Autodesk Fusion 360 part; units mm, degrees
note: some values were not read from the file. Chosen so that the rebuilt part matches the saved one: which bodies a step acts on; which face or edge a step refers to. Set by a fixed rule: which sketch regions a step uses.
(part 2 of 3)
  constraint collinear L37 L38
  constraint collinear L39 L40
  constraint coincident L41.end L43
  constraint collinear L41 L42
  constraint coincident L43.end L113
  constraint collinear L43 L44
  constraint collinear L45 L46
  constraint collinear L47 L48
  constraint coincident L50.start L55
  constraint collinear L49 L50
  constraint coincident L52.start L53
  constraint collinear L51 L52
  constraint collinear L53 L54
  constraint collinear L55 L56
  constraint coincident L58.start L59
  constraint collinear L57 L58
  constraint collinear L59 L60
  constraint coincident L62.start L111
  constraint collinear L61 L62
  constraint collinear L63 L64
  constraint coincident L65.end L67
  constraint collinear L65 L66
  constraint coincident L67.end L71
  constraint collinear L67 L68
  constraint collinear L69 L70
  constraint collinear L71 L72
  constraint collinear L73 L74
  constraint coincident L76.start L81
  constraint collinear L75 L76
  constraint coincident L78.start L79
  constraint collinear L77 L78
  constraint collinear L79 L80
  constraint collinear L81 L82
  constraint coincident L84.start L89
  constraint collinear L83 L84
  constraint coincident L86.start L109
  constraint collinear L85 L86
  constraint collinear L87 L88
  constraint collinear L89 L90
  constraint coincident L91.end L95
  constraint collinear L91 L92
  constraint collinear L93 L94
  constraint coincident L95.end L99
  constraint collinear L95 L96
  constraint collinear L97 L98
  constraint collinear L99 L100
  constraint coincident L102.start L107
  constraint collinear L101 L102
  constraint coincident L104.start L105
  constraint collinear L103 L104
  constraint collinear L105 L106
  constraint collinear L107 L108
  constraint collinear L109 L110
  constraint collinear L111 L112
  constraint collinear L113 L114
  constraint perpendicular L35 L115
  constraint perpendicular L36 L116
  constraint collinear L341 L342
  constraint coincident L344.start L349
  constraint collinear L343 L344
  constraint coincident L346.start L347
  constraint collinear L345 L346
  constraint collinear L347 L348
  constraint collinear L349 L350
  constraint coincident L351.end L355
  constraint collinear L351 L352
  constraint collinear L353 L354
  constraint coincident L355.end L367
  constraint collinear L355 L356
  constraint coincident L358.start L365
  constraint collinear L357 L358
  constraint coincident L360.start L361
  constraint collinear L359 L360
  constraint coincident A101.end L361
  constraint collinear L361 L362
  constraint collinear L363 L364
  constraint collinear L365 L366
  constraint collinear L367 L368
  constraint coincident L370.start L375
  constraint collinear L369 L370
  constraint coincident L372.start L373
  constraint collinear L371 L372
  constraint collinear L373 L374
  constraint collinear L375 L376
  constraint collinear L377 L378
  constraint coincident L379.end L383
  constraint collinear L379 L380
  constraint coincident L381.end L385
  constraint collinear L381 L382
  constraint collinear L383 L384
  constraint collinear L385 L386
  constraint collinear L387 L388
  constraint coincident L388.start L395
  constraint collinear L389 L390
  constraint coincident L392.start L393
  constraint collinear L391 L392
  constraint collinear L393 L394
  constraint collinear L395 L396
  constraint coincident L398.start L403
  constraint collinear L397 L398
  constraint coincident L400.start L401
  constraint collinear L399 L400
  constraint collinear L401 L402
  constraint collinear L403 L404
  constraint coincident L405.end L409
  constraint collinear L405 L406
  constraint collinear L407 L408
  constraint coincident L409.end L413
  constraint collinear L409 L410
  constraint collinear L411 L412
  constraint collinear L413 L414
  constraint coincident L416.start L423
  constraint collinear L415 L416
  constraint coincident L418.start L421
  constraint collinear L417 L418
  constraint collinear L419 L420
  constraint collinear L421 L422
  constraint collinear L423 L424
  measures "d74" distance of L342.end L352.end
  measures "d82" distance of L341 L355
  measures "d88" diameter of A100
  measures "d89" diameter of A99
  measures "d93" distance of L349 L367
  measures "d95" distance of L341.start L342.end
  measures "d98" distance of A100.centre L367
  measures "d103" distance of L341 L343
  measures "d104" diameter of A97
  measures "d105" diameter of A98
  measures "d106" diameter of A96
  measures "d107" distance of A96.centre L341
  measures "d113" distance of L3.start L3.end
move_body "Sposta4" bodies 1 to x (1, 0, 0) y (0, 1, 0) z (0, 0, 1) at (-120, 0, 0) in component "Cubo"
extrude "Estrusione10" cut sketch "Schizzo14" against normal blind 10 bodies 2 in component "Cubo"
fillet "Raccordo2" radius 2 4 edges at (86, 4, 13.5) (86, 86, 13.5) (4, 4, 13.5) (4, 86, 13.5) on bodies 2 in component "Cubo"
sketch "Schizzo17" plane through (0, 0, 16) normal (0, 0, 1) x (-1, 0, 0) in component "Cubo"
  line L0 (-47.5456, -19.25) -> (-48.649, -19.25)
  arc A0 (-48.649, -18.05) -> (-48.649, -19.25) centre (-49.7456, -18.65) ccw
  line L1 (-48.649, -18.05) -> (-47.5456, -18.05)
  line L2 (-47.5456, -18.05) -> (-47.5456, -12.5)
  line L3 (-47.5456, -12.5) -> (-46.2956, -12.5)
  line L4 (-46.2956, -12.5) -> (-46.2956, -10.9)
  line L5 (-46.2956, -10.9) -> (-48.649, -10.9)
  arc A1 (-48.649, -9.7) -> (-48.649, -10.9) centre (-49.7456, -10.3) ccw
  line L6 (-48.649, -9.7) -> (-46.2956, -9.7)
  line L7 (-46.2956, -9.7) -> (-46.2956, -8.9715)
  arc A2 (-43.6956, -8.9715) -> (-46.2956, -8.9715) centre (-44.9956, -7.8) ccw
  line L8 (-43.6956, -8.9715) -> (-43.6956, -9.7)
  line L9 (-43.6956, -9.7) -> (-41.3421, -9.7)
  arc A3 (-41.3421, -10.9) -> (-41.3421, -9.7) centre (-40.2456, -10.3) ccw
  line L10 (-41.3421, -10.9) -> (-43.6956, -10.9)
  line L11 (-43.6956, -10.9) -> (-43.6956, -12.5)
  line L12 (-43.6956, -12.5) -> (-42.4456, -12.5)
  line L13 (-42.4456, -12.5) -> (-42.4456, -18.05)
  line L14 (-42.4456, -18.05) -> (-41.3421, -18.05)
  arc A4 (-41.3421, -19.25) -> (-41.3421, -18.05) centre (-40.2456, -18.65) ccw
  line L15 (-41.3421, -19.25) -> (-42.4456, -19.25)
  line L16 (-42.4456, -19.25) -> (-42.4456, -24.8)
  line L17 (-42.4456, -24.8) -> (-43.6956, -24.8)
  line L18 (-43.6956, -24.8) -> (-43.6956, -26.4)
  line L19 (-43.6956, -26.4) -> (-41.3421, -26.4)
  arc A5 (-41.3421, -27.6) -> (-41.3421, -26.4) centre (-40.2456, -27) ccw
  line L20 (-41.3421, -27.6) -> (-43.6956, -27.6)
  line L21 (-43.6956, -27.6) -> (-43.6956, -28.3285)
  arc A6 (-46.2956, -28.3285) -> (-43.6956, -28.3285) centre (-44.9956, -29.5) ccw
  line L22 (-46.2956, -28.3285) -> (-46.2956, -27.6)
  line L23 (-46.2956, -27.6) -> (-48.649, -27.6)
  arc A7 (-48.649, -26.4) -> (-48.649, -27.6) centre (-49.7456, -27) ccw
  line L24 (-48.649, -26.4) -> (-46.2956, -26.4)
  line L25 (-46.2956, -26.4) -> (-46.2956, -24.8)
  line L26 (-46.2956, -24.8) -> (-47.5456, -24.8)
  line L27 (-47.5456, -24.8) -> (-47.5456, -19.25)
  arc A8 (-27.7171, -37.25) -> (-27.7171, -36.05) centre (-26.6206, -36.65) ccw
  line L28 (-27.7171, -37.25) -> (-30.0706, -37.25)
  line L29 (-30.0706, -37.25) -> (-30.0706, -38.85)
  line L30 (-30.0706, -38.85) -> (-28.8206, -38.85)
  line L31 (-28.8206, -38.85) -> (-28.8206, -44.4)
  line L32 (-28.8206, -44.4) -> (-27.7171, -44.4)
  arc A9 (-27.7171, -45.6) -> (-27.7171, -44.4) centre (-26.6206, -45) ccw
  line L33 (-27.7171, -45.6) -> (-28.8206, -45.6)
  line L34 (-28.8206, -45.6) -> (-28.8206, -51.15)
  line L35 (-28.8206, -51.15) -> (-30.0706, -51.15)
  line L36 (-30.0706, -51.15) -> (-30.0706, -52.75)
  line L37 (-30.0706, -52.75) -> (-27.7171, -52.75)
  arc A10 (-27.7171, -53.95) -> (-27.7171, -52.75) centre (-26.6206, -53.35) ccw
  line L38 (-27.7171, -53.95) -> (-30.0706, -53.95)
  line L39 (-30.0706, -53.95) -> (-30.0706, -54.6785)
  arc A11 (-32.6706, -54.6785) -> (-30.0706, -54.6785) centre (-31.3706, -55.85) ccw
  line L40 (-32.6706, -54.6785) -> (-32.6706, -53.95)
  line L41 (-32.6706, -53.95) -> (-35.024, -53.95)
  arc A12 (-35.024, -52.75) -> (-35.024, -53.95) centre (-36.1206, -53.35) ccw
  line L42 (-35.024, -52.75) -> (-32.6706, -52.75)
  line L43 (-32.6706, -52.75) -> (-32.6706, -51.15)
  line L44 (-32.6706, -51.15) -> (-33.9206, -51.15)
  line L45 (-33.9206, -51.15) -> (-33.9206, -45.6)
  line L46 (-33.9206, -45.6) -> (-35.024, -45.6)
  arc A13 (-35.024, -44.4) -> (-35.024, -45.6) centre (-36.1206, -45) ccw
  line L47 (-35.024, -44.4) -> (-33.9206, -44.4)
  line L48 (-33.9206, -44.4) -> (-33.9206, -38.85)
  line L49 (-33.9206, -38.85) -> (-32.6706, -38.85)
  line L50 (-32.6706, -38.85) -> (-32.6706, -37.25)
  line L51 (-32.6706, -37.25) -> (-35.024, -37.25)
  arc A14 (-35.024, -36.05) -> (-35.024, -37.25) centre (-36.1206, -36.65) ccw
  line L52 (-35.024, -36.05) -> (-32.6706, -36.05)
  line L53 (-32.6706, -36.05) -> (-32.6706, -35.3215)
  arc A15 (-30.0706, -35.3215) -> (-32.6706, -35.3215) centre (-31.3706, -34.15) ccw
  line L54 (-30.0706, -35.3215) -> (-30.0706, -36.05)
  line L55 (-30.0706, -36.05) -> (-27.7171, -36.05)
  line L56 (-70.9456, -79.1) -> (-68.5921, -79.1)
  arc A16 (-68.5921, -80.3) -> (-68.5921, -79.1) centre (-67.4956, -79.7) ccw
  line L57 (-68.5921, -80.3) -> (-70.9456, -80.3)
  line L58 (-70.9456, -80.3) -> (-70.9456, -81.0285)
  arc A17 (-73.5456, -81.0285) -> (-70.9456, -81.0285) centre (-72.2456, -82.2) ccw
  line L59 (-73.5456, -81.0285) -> (-73.5456, -80.3)
  line L60 (-73.5456, -80.3) -> (-75.899, -80.3)
  arc A18 (-75.899, -79.1) -> (-75.899, -80.3) centre (-76.9956, -79.7) ccw
  line L61 (-75.899, -79.1) -> (-73.5456, -79.1)
  line L62 (-73.5456, -79.1) -> (-73.5456, -77.5)
  line L63 (-73.5456, -77.5) -> (-74.7956, -77.5)
  line L64 (-74.7956, -77.5) -> (-74.7956, -71.95)
  line L65 (-74.7956, -71.95) -> (-75.899, -71.95)
  arc A19 (-75.899, -70.75) -> (-75.899, -71.95) centre (-76.9956, -71.35) ccw
  line L66 (-75.899, -70.75) -> (-74.7956, -70.75)
  line L67 (-74.7956, -70.75) -> (-74.7956, -65.2)
  line L68 (-74.7956, -65.2) -> (-73.5456, -65.2)
  line L69 (-73.5456, -65.2) -> (-73.5456, -63.6)
  line L70 (-73.5456, -63.6) -> (-75.899, -63.6)
  arc A20 (-75.899, -62.4) -> (-75.899, -63.6) centre (-76.9956, -63) ccw
  line L71 (-75.899, -62.4) -> (-73.5456, -62.4)
  line L72 (-73.5456, -62.4) -> (-73.5456, -61.6715)
  arc A21 (-70.9456, -61.6715) -> (-73.5456, -61.6715) centre (-72.2456, -60.5) ccw
  line L73 (-70.9456, -61.6715) -> (-70.9456, -62.4)
  line L74 (-70.9456, -62.4) -> (-68.5921, -62.4)
  arc A22 (-68.5921, -63.6) -> (-68.5921, -62.4) centre (-67.4956, -63) ccw
  line L75 (-68.5921, -63.6) -> (-70.9456, -63.6)
  line L76 (-70.9456, -63.6) -> (-70.9456, -65.2)
  line L77 (-70.9456, -65.2) -> (-69.6956, -65.2)
  line L78 (-69.6956, -65.2) -> (-69.6956, -70.75)
  line L79 (-69.6956, -70.75) -> (-68.5921, -70.75)
  arc A23 (-68.5921, -71.95) -> (-68.5921, -70.75) centre (-67.4956, -71.35) ccw
  line L80 (-68.5921, -71.95) -> (-69.6956, -71.95)
  line L81 (-69.6956, -71.95) -> (-69.6956, -77.5)
  line L82 (-69.6956, -77.5) -> (-70.9456, -77.5)
  line L83 (-70.9456, -77.5) -> (-70.9456, -79.1)
  line L84 (-15.1956, -70.75) -> (-14.0921, -70.75)
  arc A24 (-14.0921, -71.95) -> (-14.0921, -70.75) centre (-12.9956, -71.35) ccw
  line L85 (-14.0921, -71.95) -> (-15.1956, -71.95)
  line L86 (-15.1956, -71.95) -> (-15.1956, -77.5)
  line L87 (-15.1956, -77.5) -> (-16.4456, -77.5)
  line L88 (-16.4456, -77.5) -> (-16.4456, -79.1)
  line L89 (-16.4456, -79.1) -> (-14.0921, -79.1)
  arc A25 (-14.0921, -80.3) -> (-14.0921, -79.1) centre (-12.9956, -79.7) ccw
  line L90 (-14.0921, -80.3) -> (-16.4456, -80.3)
  line L91 (-16.4456, -80.3) -> (-16.4456, -81.0285)
  arc A26 (-19.0456, -81.0285) -> (-16.4456, -81.0285) centre (-17.7456, -82.2) ccw
  line L92 (-19.0456, -81.0285) -> (-19.0456, -80.3)
  line L93 (-19.0456, -80.3) -> (-21.399, -80.3)
  arc A27 (-21.399, -79.1) -> (-21.399, -80.3) centre (-22.4956, -79.7) ccw
  line L94 (-21.399, -79.1) -> (-19.0456, -79.1)
  line L95 (-19.0456, -79.1) -> (-19.0456, -77.5)
  line L96 (-19.0456, -77.5) -> (-20.2956, -77.5)
  line L97 (-20.2956, -77.5) -> (-20.2956, -71.95)
  line L98 (-20.2956, -71.95) -> (-21.399, -71.95)
  arc A28 (-21.399, -70.75) -> (-21.399, -71.95) centre (-22.4956, -71.35) ccw
  line L99 (-21.399, -70.75) -> (-20.2956, -70.75)
  line L100 (-20.2956, -70.75) -> (-20.2956, -65.2)
  line L101 (-20.2956, -65.2) -> (-19.0456, -65.2)
  line L102 (-19.0456, -65.2) -> (-19.0456, -63.6)
  line L103 (-19.0456, -63.6) -> (-21.399, -63.6)
  arc A29 (-21.399, -62.4) -> (-21.399, -63.6) centre (-22.4956, -63) ccw
  line L104 (-21.399, -62.4) -> (-19.0456, -62.4)
  line L105 (-19.0456, -62.4) -> (-19.0456, -61.6715)
  arc A30 (-16.4456, -61.6715) -> (-19.0456, -61.6715) centre (-17.7456, -60.5) ccw
  line L106 (-16.4456, -61.6715) -> (-16.4456, -62.4)
  line L107 (-16.4456, -62.4) -> (-14.0921, -62.4)
  arc A31 (-14.0921, -63.6) -> (-14.0921, -62.4) centre (-12.9956, -63) ccw
  line L108 (-14.0921, -63.6) -> (-16.4456, -63.6)
  line L109 (-16.4456, -63.6) -> (-16.4456, -65.2)
  line L110 (-16.4456, -65.2) -> (-15.1956, -65.2)
  line L111 (-15.1956, -65.2) -> (-15.1956, -70.75)
  line L112 (-57.3206, -62.4) -> (-54.9671, -62.4)
  arc A32 (-54.9671, -63.6) -> (-54.9671, -62.4) centre (-53.8706, -63) ccw
  line L113 (-54.9671, -63.6) -> (-57.3206, -63.6)
  line L114 (-57.3206, -63.6) -> (-57.3206, -65.2)
  line L115 (-57.3206, -65.2) -> (-56.0706, -65.2)
  line L116 (-56.0706, -65.2) -> (-56.0706, -70.75)
  line L117 (-56.0706, -70.75) -> (-54.9671, -70.75)
  arc A33 (-54.9671, -71.95) -> (-54.9671, -70.75) centre (-53.8706, -71.35) ccw
  line L118 (-54.9671, -71.95) -> (-56.0706, -71.95)
  line L119 (-56.0706, -71.95) -> (-56.0706, -77.5)
  line L120 (-56.0706, -77.5) -> (-57.3206, -77.5)
  line L121 (-57.3206, -77.5) -> (-57.3206, -79.1)
  line L122 (-57.3206, -79.1) -> (-54.9671, -79.1)
  arc A34 (-54.9671, -80.3) -> (-54.9671, -79.1) centre (-53.8706, -79.7) ccw
  line L123 (-54.9671, -80.3) -> (-57.3206, -80.3)
  line L124 (-57.3206, -80.3) -> (-57.3206, -81.0285)
  arc A35 (-59.9206, -81.0285) -> (-57.3206, -81.0285) centre (-58.6206, -82.2) ccw
  line L125 (-59.9206, -81.0285) -> (-59.9206, -80.3)
  line L126 (-59.9206, -80.3) -> (-62.274, -80.3)
  arc A36 (-62.274, -79.1) -> (-62.274, -80.3) centre (-63.3706, -79.7) ccw
  line L127 (-62.274, -79.1) -> (-59.9206, -79.1)
  line L128 (-59.9206, -79.1) -> (-59.9206, -77.5)
  line L129 (-59.9206, -77.5) -> (-61.1706, -77.5)
  line L130 (-61.1706, -77.5) -> (-61.1706, -71.95)
  line L131 (-61.1706, -71.95) -> (-62.274, -71.95)
  arc A37 (-62.274, -70.75) -> (-62.274, -71.95) centre (-63.3706, -71.35) ccw
  line L132 (-62.274, -70.75) -> (-61.1706, -70.75)
  line L133 (-61.1706, -70.75) -> (-61.1706, -65.2)
  line L134 (-61.1706, -65.2) -> (-59.9206, -65.2)
  line L135 (-59.9206, -65.2) -> (-59.9206, -63.6)
  line L136 (-59.9206, -63.6) -> (-62.274, -63.6)
  arc A38 (-62.274, -62.4) -> (-62.274, -63.6) centre (-63.3706, -63) ccw
  line L137 (-62.274, -62.4) -> (-59.9206, -62.4)
  line L138 (-59.9206, -62.4) -> (-59.9206, -61.6715)
  arc A39 (-57.3206, -61.6715) -> (-59.9206, -61.6715) centre (-58.6206, -60.5) ccw
  line L139 (-57.3206, -61.6715) -> (-57.3206, -62.4)
  line L140 (-47.5456, -45.6) -> (-48.649, -45.6)
  arc A40 (-48.649, -44.4) -> (-48.649, -45.6) centre (-49.7456, -45) ccw
  line L141 (-48.649, -44.4) -> (-47.5456, -44.4)
  line L142 (-47.5456, -44.4) -> (-47.5456, -38.85)
  line L143 (-47.5456, -38.85) -> (-46.2956, -38.85)
  line L144 (-46.2956, -38.85) -> (-46.2956, -37.25)
  line L145 (-46.2956, -37.25) -> (-48.649, -37.25)
  arc A41 (-48.649, -36.05) -> (-48.649, -37.25) centre (-49.7456, -36.65) ccw
  line L146 (-48.649, -36.05) -> (-46.2956, -36.05)
  line L147 (-46.2956, -36.05) -> (-46.2956, -35.3215)
  arc A42 (-43.6956, -35.3215) -> (-46.2956, -35.3215) centre (-44.9956, -34.15) ccw
  line L148 (-43.6956, -35.3215) -> (-43.6956, -36.05)
  line L149 (-43.6956, -36.05) -> (-41.3421, -36.05)
  arc A43 (-41.3421, -37.25) -> (-41.3421, -36.05) centre (-40.2456, -36.65) ccw
  line L150 (-41.3421, -37.25) -> (-43.6956, -37.25)
  line L151 (-43.6956, -37.25) -> (-43.6956, -38.85)
  line L152 (-43.6956, -38.85) -> (-42.4456, -38.85)
  line L153 (-42.4456, -38.85) -> (-42.4456, -44.4)
  line L154 (-42.4456, -44.4) -> (-41.3421, -44.4)
  arc A44 (-41.3421, -45.6) -> (-41.3421, -44.4) centre (-40.2456, -45) ccw
  line L155 (-41.3421, -45.6) -> (-42.4456, -45.6)
  line L156 (-42.4456, -45.6) -> (-42.4456, -51.15)
  line L157 (-42.4456, -51.15) -> (-43.6956, -51.15)
  line L158 (-43.6956, -51.15) -> (-43.6956, -52.75)
  line L159 (-43.6956, -52.75) -> (-41.3421, -52.75)
  arc A45 (-41.3421, -53.95) -> (-41.3421, -52.75) centre (-40.2456, -53.35) ccw
  line L160 (-41.3421, -53.95) -> (-43.6956, -53.95)
  line L161 (-43.6956, -53.95) -> (-43.6956, -54.6785)
  arc A46 (-46.2956, -54.6785) -> (-43.6956, -54.6785) centre (-44.9956, -55.85) ccw
  line L162 (-46.2956, -54.6785) -> (-46.2956, -53.95)
  line L163 (-46.2956, -53.95) -> (-48.649, -53.95)
  arc A47 (-48.649, -52.75) -> (-48.649, -53.95) centre (-49.7456, -53.35) ccw
  line L164 (-48.649, -52.75) -> (-46.2956, -52.75)
  line L165 (-46.2956, -52.75) -> (-46.2956, -51.15)
  line L166 (-46.2956, -51.15) -> (-47.5456, -51.15)
  line L167 (-47.5456, -51.15) -> (-47.5456, -45.6)
  arc A48 (-27.7171, -10.9) -> (-27.7171, -9.7) centre (-26.6206, -10.3) ccw
  line L168 (-27.7171, -10.9) -> (-30.0706, -10.9)
  line L169 (-30.0706, -10.9) -> (-30.0706, -12.5)
  line L170 (-30.0706, -12.5) -> (-28.8206, -12.5)
  line L171 (-28.8206, -12.5) -> (-28.8206, -18.05)
  line L172 (-28.8206, -18.05) -> (-27.7171, -18.05)
  arc A49 (-27.7171, -19.25) -> (-27.7171, -18.05) centre (-26.6206, -18.65) ccw
  line L173 (-27.7171, -19.25) -> (-28.8206, -19.25)
  line L174 (-28.8206, -19.25) -> (-28.8206, -24.8)
  line L175 (-28.8206, -24.8) -> (-30.0706, -24.8)
  line L176 (-30.0706, -24.8) -> (-30.0706, -26.4)
  line L177 (-30.0706, -26.4) -> (-27.7171, -26.4)
  arc A50 (-27.7171, -27.6) -> (-27.7171, -26.4) centre (-26.6206, -27) ccw
  line L178 (-27.7171, -27.6) -> (-30.0706, -27.6)
  line L179 (-30.0706, -27.6) -> (-30.0706, -28.3285)
  arc A51 (-32.6706, -28.3285) -> (-30.0706, -28.3285) centre (-31.3706, -29.5) ccw
  line L180 (-32.6706, -28.3285) -> (-32.6706, -27.6)
  line L181 (-32.6706, -27.6) -> (-35.024, -27.6)
  arc A52 (-35.024, -26.4) -> (-35.024, -27.6) centre (-36.1206, -27) ccw
  line L182 (-35.024, -26.4) -> (-32.6706, -26.4)
  line L183 (-32.6706, -26.4) -> (-32.6706, -24.8)
  line L184 (-32.6706, -24.8) -> (-33.9206, -24.8)
  line L185 (-33.9206, -24.8) -> (-33.9206, -19.25)
  line L186 (-33.9206, -19.25) -> (-35.024, -19.25)
  arc A53 (-35.024, -18.05) -> (-35.024, -19.25) centre (-36.1206, -18.65) ccw
  line L187 (-35.024, -18.05) -> (-33.9206, -18.05)
  line L188 (-33.9206, -18.05) -> (-33.9206, -12.5)
  line L189 (-33.9206, -12.5) -> (-32.6706, -12.5)
  line L190 (-32.6706, -12.5) -> (-32.6706, -10.9)
  line L191 (-32.6706, -10.9) -> (-35.024, -10.9)
  arc A54 (-35.024, -9.7) -> (-35.024, -10.9) centre (-36.1206, -10.3) ccw
  line L192 (-35.024, -9.7) -> (-32.6706, -9.7)
  line L193 (-32.6706, -9.7) -> (-32.6706, -8.9715)
  arc A55 (-30.0706, -8.9715) -> (-32.6706, -8.9715) centre (-31.3706, -7.8) ccw
  line L194 (-30.0706, -8.9715) -> (-30.0706, -9.7)
  line L195 (-30.0706, -9.7) -> (-27.7171, -9.7)
  line L196 (-59.9206, -27.6) -> (-62.274, -27.6)
  arc A56 (-62.274, -26.4) -> (-62.274, -27.6) centre (-63.3706, -27) ccw
  line L197 (-62.274, -26.4) -> (-59.9206, -26.4)
  line L198 (-59.9206, -26.4) -> (-59.9206, -24.8)
  line L199 (-59.9206, -24.8) -> (-61.1706, -24.8)
  line L200 (-61.1706, -24.8) -> (-61.1706, -19.25)
  line L201 (-61.1706, -19.25) -> (-62.274, -19.25)
  arc A57 (-62.274, -18.05) -> (-62.274, -19.25) centre (-63.3706, -18.65) ccw
  line L202 (-62.274, -18.05) -> (-61.1706, -18.05)
  line L203 (-61.1706, -18.05) -> (-61.1706, -12.5)
  line L204 (-61.1706, -12.5) -> (-59.9206, -12.5)
  line L205 (-59.9206, -12.5) -> (-59.9206, -10.9)
  line L206 (-59.9206, -10.9) -> (-62.274, -10.9)
  arc A58 (-62.274, -9.7) -> (-62.274, -10.9) centre (-63.3706, -10.3) ccw
  line L207 (-62.274, -9.7) -> (-59.9206, -9.7)
  line L208 (-59.9206, -9.7) -> (-59.9206, -8.9715)
  arc A59 (-57.3206, -8.9715) -> (-59.9206, -8.9715) centre (-58.6206, -7.8) ccw
  line L209 (-57.3206, -8.9715) -> (-57.3206, -9.7)
  line L210 (-57.3206, -9.7) -> (-54.9671, -9.7)
  arc A60 (-54.9671, -10.9) -> (-54.9671, -9.7) centre (-53.8706, -10.3) ccw
  line L211 (-54.9671, -10.9) -> (-57.3206, -10.9)
  line L212 (-57.3206, -10.9) -> (-57.3206, -12.5)
  line L213 (-57.3206, -12.5) -> (-56.0706, -12.5)
  line L214 (-56.0706, -12.5) -> (-56.0706, -18.05)
  line L215 (-56.0706, -18.05) -> (-54.9671, -18.05)
  arc A61 (-54.9671, -19.25) -> (-54.9671, -18.05) centre (-53.8706, -18.65) ccw
  line L216 (-54.9671, -19.25) -> (-56.0706, -19.25)
  line L217 (-56.0706, -19.25) -> (-56.0706, -24.8)
  line L218 (-56.0706, -24.8) -> (-57.3206, -24.8)
  line L219 (-57.3206, -24.8) -> (-57.3206, -26.4)
  line L220 (-57.3206, -26.4) -> (-54.9671, -26.4)
  arc A62 (-54.9671, -27.6) -> (-54.9671, -26.4) centre (-53.8706, -27) ccw
  line L221 (-54.9671, -27.6) -> (-57.3206, -27.6)
  line L222 (-57.3206, -27.6) -> (-57.3206, -28.3285)
  arc A63 (-59.9206, -28.3285) -> (-57.3206, -28.3285) centre (-58.6206, -29.5) ccw
  line L223 (-59.9206, -28.3285) -> (-59.9206, -27.6)
  line L224 (-16.4456, -36.05) -> (-14.0921, -36.05)
  arc A64 (-14.0921, -37.25) -> (-14.0921, -36.05) centre (-12.9956, -36.65) ccw
  line L225 (-14.0921, -37.25) -> (-16.4456, -37.25)
  line L226 (-16.4456, -37.25) -> (-16.4456, -38.85)
  line L227 (-16.4456, -38.85) -> (-15.1956, -38.85)
  line L228 (-15.1956, -38.85) -> (-15.1956, -44.4)
  line L229 (-15.1956, -44.4) -> (-14.0921, -44.4)
  arc A65 (-14.0921, -45.6) -> (-14.0921, -44.4) centre (-12.9956, -45) ccw
  line L230 (-14.0921, -45.6) -> (-15.1956, -45.6)
  line L231 (-15.1956, -45.6) -> (-15.1956, -51.15)
  line L232 (-15.1956, -51.15) -> (-16.4456, -51.15)
  line L233 (-16.4456, -51.15) -> (-16.4456, -52.75)
  line L234 (-16.4456, -52.75) -> (-14.0921, -52.75)
  arc A66 (-14.0921, -53.95) -> (-14.0921, -52.75) centre (-12.9956, -53.35) ccw
  line L235 (-14.0921, -53.95) -> (-16.4456, -53.95)
  line L236 (-16.4456, -53.95) -> (-16.4456, -54.6785)
  arc A67 (-19.0456, -54.6785) -> (-16.4456, -54.6785) centre (-17.7456, -55.85) ccw
  line L237 (-19.0456, -54.6785) -> (-19.0456, -53.95)
  line L238 (-19.0456, -53.95) -> (-21.399, -53.95)
  arc A68 (-21.399, -52.75) -> (-21.399, -53.95) centre (-22.4956, -53.35) ccw
  line L239 (-21.399, -52.75) -> (-19.0456, -52.75)
  line L240 (-19.0456, -52.75) -> (-19.0456, -51.15)
  line L241 (-19.0456, -51.15) -> (-20.2956, -51.15)
  line L242 (-20.2956, -51.15) -> (-20.2956, -45.6)
  line L243 (-20.2956, -45.6) -> (-21.399, -45.6)
  arc A69 (-21.399, -44.4) -> (-21.399, -45.6) centre (-22.4956, -45) ccw
  line L244 (-21.399, -44.4) -> (-20.2956, -44.4)
  line L245 (-20.2956, -44.4) -> (-20.2956, -38.85)
  line L246 (-20.2956, -38.85) -> (-19.0456, -38.85)
  line L247 (-19.0456, -38.85) -> (-19.0456, -37.25)
  line L248 (-19.0456, -37.25) -> (-21.399, -37.25)
  arc A70 (-21.399, -36.05) -> (-21.399, -37.25) centre (-22.4956, -36.65) ccw
  line L249 (-21.399, -36.05) -> (-19.0456, -36.05)
  line L250 (-19.0456, -36.05) -> (-19.0456, -35.3215)
  arc A71 (-16.4456, -35.3215) -> (-19.0456, -35.3215) centre (-17.7456, -34.15) ccw
  line L251 (-16.4456, -35.3215) -> (-16.4456, -36.05)
  arc A72 (-68.5921, -37.25) -> (-68.5921, -36.05) centre (-67.4956, -36.65) ccw
  line L252 (-68.5921, -37.25) -> (-70.9456, -37.25)
  line L253 (-70.9456, -37.25) -> (-70.9456, -38.85)
  line L254 (-70.9456, -38.85) -> (-69.6956, -38.85)
  line L255 (-69.6956, -38.85) -> (-69.6956, -44.4)
  line L256 (-69.6956, -44.4) -> (-68.5921, -44.4)
  arc A73 (-68.5921, -45.6) -> (-68.5921, -44.4) centre (-67.4956, -45) ccw
  line L257 (-68.5921, -45.6) -> (-69.6956, -45.6)
  line L258 (-69.6956, -45.6) -> (-69.6956, -51.15)
  line L259 (-69.6956, -51.15) -> (-70.9456, -51.15)
  line L260 (-70.9456, -51.15) -> (-70.9456, -52.75)
  line L261 (-70.9456, -52.75) -> (-68.5921, -52.75)
  arc A74 (-68.5921, -53.95) -> (-68.5921, -52.75) centre (-67.4956, -53.35) ccw
  line L262 (-68.5921, -53.95) -> (-70.9456, -53.95)
  line L263 (-70.9456, -53.95) -> (-70.9456, -54.6785)
  arc A75 (-73.5456, -54.6785) -> (-70.9456, -54.6785) centre (-72.2456, -55.85) ccw
  line L264 (-73.5456, -54.6785) -> (-73.5456, -53.95)
  line L265 (-73.5456, -53.95) -> (-75.899, -53.95)
  arc A76 (-75.899, -52.75) -> (-75.899, -53.95) centre (-76.9956, -53.35) ccw
  line L266 (-75.899, -52.75) -> (-73.5456, -52.75)
  line L267 (-73.5456, -52.75) -> (-73.5456, -51.15)
  line L268 (-73.5456, -51.15) -> (-74.7956, -51.15)
  line L269 (-74.7956, -51.15) -> (-74.7956, -45.6)
  line L270 (-74.7956, -45.6) -> (-75.899, -45.6)
  arc A77 (-75.899, -44.4) -> (-75.899, -45.6) centre (-76.9956, -45) ccw
  line L271 (-75.899, -44.4) -> (-74.7956, -44.4)
  line L272 (-74.7956, -44.4) -> (-74.7956, -38.85)
  line L273 (-74.7956, -38.85) -> (-73.5456, -38.85)
  line L274 (-73.5456, -38.85) -> (-73.5456, -37.25)
  line L275 (-73.5456, -37.25) -> (-75.899, -37.25)
  arc A78 (-75.899, -36.05) -> (-75.899, -37.25) centre (-76.9956, -36.65) ccw
  line L276 (-75.899, -36.05) -> (-73.5456, -36.05)
  line L277 (-73.5456, -36.05) -> (-73.5456, -35.3215)
  arc A79 (-70.9456, -35.3215) -> (-73.5456, -35.3215) centre (-72.2456, -34.15) ccw
  line L278 (-70.9456, -35.3215) -> (-70.9456, -36.05)
  line L279 (-70.9456, -36.05) -> (-68.5921, -36.05)
  line L280 (-32.6706, -80.3) -> (-35.024, -80.3)
  arc A80 (-35.024, -79.1) -> (-35.024, -80.3) centre (-36.1206, -79.7) ccw
  line L281 (-35.024, -79.1) -> (-32.6706, -79.1)
  line L282 (-32.6706, -79.1) -> (-32.6706, -77.5)
  line L283 (-32.6706, -77.5) -> (-33.9206, -77.5)
  line L284 (-33.9206, -77.5) -> (-33.9206, -71.95)
  line L285 (-33.9206, -71.95) -> (-35.024, -71.95)
  arc A81 (-35.024, -70.75) -> (-35.024, -71.95) centre (-36.1206, -71.35) ccw
  line L286 (-35.024, -70.75) -> (-33.9206, -70.75)
  line L287 (-33.9206, -70.75) -> (-33.9206, -65.2)
  line L288 (-33.9206, -65.2) -> (-32.6706, -65.2)
  line L289 (-32.6706, -65.2) -> (-32.6706, -63.6)
  line L290 (-32.6706, -63.6) -> (-35.024, -63.6)
  arc A82 (-35.024, -62.4) -> (-35.024, -63.6) centre (-36.1206, -63) ccw
  line L291 (-35.024, -62.4) -> (-32.6706, -62.4)
  line L292 (-32.6706, -62.4) -> (-32.6706, -61.6715)
  arc A83 (-30.0706, -61.6715) -> (-32.6706, -61.6715) centre (-31.3706, -60.5) ccw
  line L293 (-30.0706, -61.6715) -> (-30.0706, -62.4)
  line L294 (-30.0706, -62.4) -> (-27.7171, -62.4)
  arc A84 (-27.7171, -63.6) -> (-27.7171, -62.4) centre (-26.6206, -63) ccw
  line L295 (-27.7171, -63.6) -> (-30.0706, -63.6)
  line L296 (-30.0706, -63.6) -> (-30.0706, -65.2)
  line L297 (-30.0706, -65.2) -> (-28.8206, -65.2)
  line L298 (-28.8206, -65.2) -> (-28.8206, -70.75)
  line L299 (-28.8206, -70.75) -> (-27.7171, -70.75)
  arc A85 (-27.7171, -71.95) -> (-27.7171, -70.75) centre (-26.6206, -71.35) ccw
  line L300 (-27.7171, -71.95) -> (-28.8206, -71.95)
  line L301 (-28.8206, -71.95) -> (-28.8206, -77.5)
  line L302 (-28.8206, -77.5) -> (-30.0706, -77.5)
  line L303 (-30.0706, -77.5) -> (-30.0706, -79.1)
  line L304 (-30.0706, -79.1) -> (-27.7171, -79.1)
  arc A86 (-27.7171, -80.3) -> (-27.7171, -79.1) centre (-26.6206, -79.7) ccw
  line L305 (-27.7171, -80.3) -> (-30.0706, -80.3)
  line L306 (-30.0706, -80.3) -> (-30.0706, -81.0285)
  arc A87 (-32.6706, -81.0285) -> (-30.0706, -81.0285) centre (-31.3706, -82.2) ccw
  line L307 (-32.6706, -81.0285) -> (-32.6706, -80.3)
  arc A88 (-46.2956, -81.0285) -> (-43.6956, -81.0285) centre (-44.9956, -82.2) ccw
  line L308 (-46.2956, -81.0285) -> (-46.2956, -80.3)
  line L309 (-46.2956, -80.3) -> (-48.649, -80.3)
  arc A89 (-48.649, -79.1) -> (-48.649, -80.3) centre (-49.7456, -79.7) ccw
  line L310 (-48.649, -79.1) -> (-46.2956, -79.1)
  line L311 (-46.2956, -79.1) -> (-46.2956, -77.5)
  line L312 (-46.2956, -77.5) -> (-47.5456, -77.5)
  line L313 (-47.5456, -77.5) -> (-47.5456, -71.95)
  line L314 (-47.5456, -71.95) -> (-48.649, -71.95)
  arc A90 (-48.649, -70.75) -> (-48.649, -71.95) centre (-49.7456, -71.35) ccw
  line L315 (-48.649, -70.75) -> (-47.5456, -70.75)
  line L316 (-47.5456, -70.75) -> (-47.5456, -65.2)
  line L317 (-47.5456, -65.2) -> (-46.2956, -65.2)
  line L318 (-46.2956, -65.2) -> (-46.2956, -63.6)
  line L319 (-46.2956, -63.6) -> (-48.649, -63.6)
  arc A91 (-48.649, -62.4) -> (-48.649, -63.6) centre (-49.7456, -63) ccw
  line L320 (-48.649, -62.4) -> (-46.2956, -62.4)
  line L321 (-46.2956, -62.4) -> (-46.2956, -61.6715)
  arc A92 (-43.6956, -61.6715) -> (-46.2956, -61.6715) centre (-44.9956, -60.5) ccw
  line L322 (-43.6956, -61.6715) -> (-43.6956, -62.4)
  line L323 (-43.6956, -62.4) -> (-41.3421, -62.4)
  arc A93 (-41.3421, -63.6) -> (-41.3421, -62.4) centre (-40.2456, -63) ccw
  line L324 (-41.3421, -63.6) -> (-43.6956, -63.6)
  line L325 (-43.6956, -63.6) -> (-43.6956, -65.2)
  line L326 (-43.6956, -65.2) -> (-42.4456, -65.2)
  line L327 (-42.4456, -65.2) -> (-42.4456, -70.75)
  line L328 (-42.4456, -70.75) -> (-41.3421, -70.75)
  arc A94 (-41.3421, -71.95) -> (-41.3421, -70.75) centre (-40.2456, -71.35) ccw
  line L329 (-41.3421, -71.95) -> (-42.4456, -71.95)
  line L330 (-42.4456, -71.95) -> (-42.4456, -77.5)
  line L331 (-42.4456, -77.5) -> (-43.6956, -77.5)
  line L332 (-43.6956, -77.5) -> (-43.6956, -79.1)
  line L333 (-43.6956, -79.1) -> (-41.3421, -79.1)
  arc A95 (-41.3421, -80.3) -> (-41.3421, -79.1) centre (-40.2456, -79.7) ccw
  line L334 (-41.3421, -80.3) -> (-43.6956, -80.3)
  line L335 (-43.6956, -80.3) -> (-43.6956, -81.0285)
  line L336 (-59.9206, -53.95) -> (-62.274, -53.95)
  arc A96 (-62.274, -52.75) -> (-62.274, -53.95) centre (-63.3706, -53.35) ccw
  line L337 (-62.274, -52.75) -> (-59.9206, -52.75)
  line L338 (-59.9206, -52.75) -> (-59.9206, -51.15)
  line L339 (-59.9206, -51.15) -> (-61.1706, -51.15)
  line L340 (-61.1706, -51.15) -> (-61.1706, -45.6)
  line L341 (-61.1706, -45.6) -> (-62.274, -45.6)
  arc A97 (-62.274, -44.4) -> (-62.274, -45.6) centre (-63.3706, -45) ccw
  line L342 (-62.274, -44.4) -> (-61.1706, -44.4)
  line L343 (-61.1706, -44.4) -> (-61.1706, -38.85)
  line L344 (-61.1706, -38.85) -> (-59.9206, -38.85)
  line L345 (-59.9206, -38.85) -> (-59.9206, -37.25)
  line L346 (-59.9206, -37.25) -> (-62.274, -37.25)
  arc A98 (-62.274, -36.05) -> (-62.274, -37.25) centre (-63.3706, -36.65) ccw
  line L347 (-62.274, -36.05) -> (-59.9206, -36.05)
  line L348 (-59.9206, -36.05) -> (-59.9206, -35.3215)
  arc A99 (-57.3206, -35.3215) -> (-59.9206, -35.3215) centre (-58.6206, -34.15) ccw
  line L349 (-57.3206, -35.3215) -> (-57.3206, -36.05)
  line L350 (-57.3206, -36.05) -> (-54.9671, -36.05)
  arc A100 (-54.9671, -37.25) -> (-54.9671, -36.05) centre (-53.8706, -36.65) ccw
  line L351 (-54.9671, -37.25) -> (-57.3206, -37.25)
  line L352 (-57.3206, -37.25) -> (-57.3206, -38.85)
  line L353 (-57.3206, -38.85) -> (-56.0706, -38.85)
  line L354 (-56.0706, -38.85) -> (-56.0706, -44.4)
  line L355 (-56.0706, -44.4) -> (-54.9671, -44.4)
  arc A101 (-54.9671, -45.6) -> (-54.9671, -44.4) centre (-53.8706, -45) ccw
  line L356 (-54.9671, -45.6) -> (-56.0706, -45.6)
  line L357 (-56.0706, -45.6) -> (-56.0706, -51.15)
  line L358 (-56.0706, -51.15) -> (-57.3206, -51.15)
  line L359 (-57.3206, -51.15) -> (-57.3206, -52.75)
  line L360 (-57.3206, -52.75) -> (-54.9671, -52.75)
  arc A102 (-54.9671, -53.95) -> (-54.9671, -52.75) centre (-53.8706, -53.35) ccw
  line L361 (-54.9671, -53.95) -> (-57.3206, -53.95)
  line L362 (-57.3206, -53.95) -> (-57.3206, -54.6785)
  arc A103 (-59.9206, -54.6785) -> (-57.3206, -54.6785) centre (-58.6206, -55.85) ccw
  line L363 (-59.9206, -54.6785) -> (-59.9206, -53.95)
  arc A104 (-21.399, -9.7) -> (-21.399, -10.9) centre (-22.4956, -10.3) ccw
  line L364 (-21.399, -9.7) -> (-19.0456, -9.7)
  line L365 (-19.0456, -9.7) -> (-19.0456, -8.9715)
  arc A105 (-16.4456, -8.9715) -> (-19.0456, -8.9715) centre (-17.7456, -7.8) ccw
  line L366 (-16.4456, -8.9715) -> (-16.4456, -9.7)
  line L367 (-16.4456, -9.7) -> (-14.0921, -9.7)
  arc A106 (-14.0921, -10.9) -> (-14.0921, -9.7) centre (-12.9956, -10.3) ccw
  line L368 (-14.0921, -10.9) -> (-16.4456, -10.9)
  line L369 (-16.4456, -10.9) -> (-16.4456, -12.5)
  line L370 (-16.4456, -12.5) -> (-15.1956, -12.5)
  line L371 (-15.1956, -12.5) -> (-15.1956, -18.05)
  line L372 (-15.1956, -18.05) -> (-14.0921, -18.05)
  arc A107 (-14.0921, -19.25) -> (-14.0921, -18.05) centre (-12.9956, -18.65) ccw
  line L373 (-14.0921, -19.25) -> (-15.1956, -19.25)
  line L374 (-15.1956, -19.25) -> (-15.1956, -24.8)
  line L375 (-15.1956, -24.8) -> (-16.4456, -24.8)
  line L376 (-16.4456, -24.8) -> (-16.4456, -26.4)
  line L377 (-16.4456, -26.4) -> (-14.0921, -26.4)
  arc A108 (-14.0921, -27.6) -> (-14.0921, -26.4) centre (-12.9956, -27) ccw
  line L378 (-14.0921, -27.6) -> (-16.4456, -27.6)
  line L379 (-16.4456, -27.6) -> (-16.4456, -28.3285)
  arc A109 (-19.0456, -28.3285) -> (-16.4456, -28.3285) centre (-17.7456, -29.5) ccw
  line L380 (-19.0456, -28.3285) -> (-19.0456, -27.6)
  line L381 (-19.0456, -27.6) -> (-21.399, -27.6)
  arc A110 (-21.399, -26.4) -> (-21.399, -27.6) centre (-22.4956, -27) ccw
  line L382 (-21.399, -26.4) -> (-19.0456, -26.4)
  line L383 (-19.0456, -26.4) -> (-19.0456, -24.8)
  line L384 (-19.0456, -24.8) -> (-20.2956, -24.8)
  line L385 (-20.2956, -24.8) -> (-20.2956, -19.25)
  line L386 (-20.2956, -19.25) -> (-21.399, -19.25)
  arc A111 (-21.399, -18.05) -> (-21.399, -19.25) centre (-22.4956, -18.65) ccw
  line L387 (-21.399, -18.05) -> (-20.2956, -18.05)
  line L388 (-20.2956, -18.05) -> (-20.2956, -12.5)
  line L389 (-20.2956, -12.5) -> (-19.0456, -12.5)
  line L390 (-19.0456, -12.5) -> (-19.0456, -10.9)
  line L391 (-19.0456, -10.9) -> (-21.399, -10.9)
  arc A112 (-68.5921, -10.9) -> (-68.5921, -9.7) centre (-67.4956, -10.3) ccw
  line L392 (-68.5921, -10.9) -> (-70.9456, -10.9)
  line L393 (-70.9456, -10.9) -> (-70.9456, -12.5)
  line L394 (-70.9456, -12.5) -> (-69.6956, -12.5)
  line L395 (-69.6956, -12.5) -> (-69.6956, -18.05)
  line L396 (-69.6956, -18.05) -> (-68.5921, -18.05)
  arc A113 (-68.5921, -19.25) -> (-68.5921, -18.05) centre (-67.4956, -18.65) ccw
  line L397 (-68.5921, -19.25) -> (-69.6956, -19.25)
  line L398 (-69.6956, -19.25) -> (-69.6956, -24.8)
  line L399 (-69.6956, -24.8) -> (-70.9456, -24.8)
  line L400 (-70.9456, -24.8) -> (-70.9456, -26.4)
  line L401 (-70.9456, -26.4) -> (-68.5921, -26.4)
  arc A114 (-68.5921, -27.6) -> (-68.5921, -26.4) centre (-67.4956, -27) ccw
  line L402 (-68.5921, -27.6) -> (-70.9456, -27.6)
  line L403 (-70.9456, -27.6) -> (-70.9456, -28.3285)
  arc A115 (-73.5456, -28.3285) -> (-70.9456, -28.3285) centre (-72.2456, -29.5) ccw
  line L404 (-73.5456, -28.3285) -> (-73.5456, -27.6)
  line L405 (-73.5456, -27.6) -> (-75.899, -27.6)
  arc A116 (-75.899, -26.4) -> (-75.899, -27.6) centre (-76.9956, -27) ccw
  line L406 (-75.899, -26.4) -> (-73.5456, -26.4)
  line L407 (-73.5456, -26.4) -> (-73.5456, -24.8)
  line L408 (-73.5456, -24.8) -> (-74.7956, -24.8)
  line L409 (-74.7956, -24.8) -> (-74.7956, -19.25)
  line L410 (-74.7956, -19.25) -> (-75.899, -19.25)
  arc A117 (-75.899, -18.05) -> (-75.899, -19.25) centre (-76.9956, -18.65) ccw
  line L411 (-75.899, -18.05) -> (-74.7956, -18.05)
  line L412 (-74.7956, -18.05) -> (-74.7956, -12.5)
  line L413 (-74.7956, -12.5) -> (-73.5456, -12.5)
  line L414 (-73.5456, -12.5) -> (-73.5456, -10.9)
  line L415 (-73.5456, -10.9) -> (-75.899, -10.9)
  arc A118 (-75.899, -9.7) -> (-75.899, -10.9) centre (-76.9956, -10.3) ccw
  line L416 (-75.899, -9.7) -> (-73.5456, -9.7)
  line L417 (-73.5456, -9.7) -> (-73.5456, -8.9715)
  arc A119 (-70.9456, -8.9715) -> (-73.5456, -8.9715) centre (-72.2456, -7.8) ccw
  line L418 (-70.9456, -8.9715) -> (-70.9456, -9.7)
  line L419 (-70.9456, -9.7) -> (-68.5921, -9.7)
  arc A120 (-6, -86) -> (-4, -84) centre (-6, -84) ccw
  line L420 (-4, -84) -> (-4, -6)
  arc A121 (-4, -6) -> (-6, -4) centre (-6, -6) ccw
  line L421 (-6, -4) -> (-84, -4)
  arc A122 (-84, -4) -> (-86, -6) centre (-84, -6) ccw
  line L422 (-86, -6) -> (-86, -84)
  arc A123 (-86, -84) -> (-84, -86) centre (-84, -84) ccw
  line L423 (-84, -86) -> (-6, -86)
  line L424 (0, -90) -> (-45, -90)
  line L425 (-45, -90) -> (-45, -95)
  line L426 (0, -90) -> (0, -45)
  line L427 (0, -45) -> (5, -45)
  circle A124 centre (-8, -82) radius 2.75
  circle A125 centre (-82, -82) radius 2.75
  circle A126 centre (-8, -8) radius 2.75
  circle A127 centre (-82, -8) radius 2.75
  dimension "d137" = 45
  dimension "d138" = 45
  dimension "d139" = 5.5
  constraint horizontal L424
  constraint perpendicular L424 L425
  constraint perpendicular L424 L426
  constraint perpendicular L426 L427
  constraint symmetric L425 A124 A125
  constraint symmetric L427 A124 A126
  constraint symmetric L427 A125 A127
  measures "d137" distance of L424.start L424.end
  measures "d138" distance of L424.start L426.end
  measures "d139" diameter of A124
extrude "Estrusione11" cut sketch "Schizzo17" against normal blind 1.5 contours A124 | A125 | A126 | A127 bodies 2 in component "Cubo"
sketch "Schizzo18" plane through (0, 0, 101) normal (0, 0, -1) x (1, 0, 0) in component "Cubo"
  line L0 (-33.5, -3.5) -> (-33.5, -86.5)
  line L1 (-33.5, -86.5) -> (-116.5, -86.5)
  line L2 (-116.5, -86.5) -> (-116.5, -3.5)
  line L3 (-116.5, -3.5) -> (-33.5, -3.5)
  arc A0 (-33, -90) -> (-30, -87) centre (-33, -87) ccw
  line L4 (-30, -87) -> (-30, -3)
  arc A1 (-30, -3) -> (-33, 0) centre (-33, -3) ccw
  line L5 (-33, 0) -> (-117, 0)
  arc A2 (-117, 0) -> (-120, -3) centre (-117, -3) ccw
  line L6 (-120, -3) -> (-120, -87)
  arc A3 (-120, -87) -> (-117, -90) centre (-117, -87) ccw
  line L7 (-117, -90) -> (-33, -90)
  line L8 (-116.5, -3.5) -> (-111.2322, -3.5)
  line L9 (-116.5, -12) -> (-116.5, -3.5)
  circle A4 centre (-112, -8) radius 2.75
  line L10 (-75, 0) -> (-75, 6)
  line L11 (-120, -45) -> (-130, -45)
  line L12 (-33.5, -3.5) -> (-42, -3.5)
  line L13 (-42, -3.5) -> (-42, -12)
  line L14 (-42, -12) -> (-33.5, -12)
  line L15 (-33.5, -12) -> (-33.5, -3.5)
  line L16 (-33.5, -86.5) -> (-42, -86.5)
  line L17 (-42, -86.5) -> (-42, -78)
  line L18 (-42, -78) -> (-33.5, -78)
  line L19 (-33.5, -78) -> (-33.5, -86.5)
  line L20 (-116.5, -86.5) -> (-108, -86.5)
  line L21 (-116.5, -78) -> (-116.5, -86.5)
  arc A5 (-116.5, -13.5) -> (-106.5, -3.5) centre (-116.5, -3.5) ccw
  arc A6 (-43.5, -3.5) -> (-33.5, -13.5) centre (-33.5, -3.5) ccw
  arc A7 (-33.5, -76.5) -> (-43.5, -86.5) centre (-33.5, -86.5) ccw
  arc A8 (-106.5, -86.5) -> (-116.5, -76.5) centre (-116.5, -86.5) ccw
  dimension "d146" = 5.5
  dimension "d147" = 8
  dimension "d148" = 8
  dimension "d151" = 8.5
  dimension "d152" = 8.5
  dimension "d153" = 8.5
  dimension "d154" = 8.5
  dimension "d155" = 8.5
  dimension "d156" = 8.5
  dimension "d201" = 20
  dimension "d202" = 20
  dimension "d203" = 20
  dimension "d204" = 20
  constraint horizontal L8
  constraint vertical L9
  constraint coincident L2.end L3.start
  constraint midpoint L5 L10.start
  constraint perpendicular L5 L10
  constraint midpoint L6 L11.start
  constraint perpendicular L6 L11
  constraint horizontal L12
  constraint vertical L13
  constraint horizontal L14
  constraint vertical L15
  constraint coincident L0.start L3.end
  constraint horizontal L16
  constraint vertical L17
  constraint horizontal L18
  constraint vertical L19
  constraint coincident L0.end L1.start
  constraint horizontal L20
  constraint vertical L21
  constraint coincident L1.end L2.start
  constraint coincident L3 A5.end
  constraint coincident L2 A5.start
  constraint coincident L3 A6.start
  constraint coincident L0 A6.end
  constraint coincident L0 A7.start
  constraint coincident L1 A7.end
  constraint coincident L2 A8.end
  constraint coincident L1 A8.start
  measures "d146" diameter of A4
  measures "d147" distance of L5 A4.centre
  measures "d148" distance of L6 A4.centre
  measures "d151" distance of L0.start L12.end
  measures "d152" distance of L0.start L14.end
  measures "d153" distance of L0.end L16.end
  measures "d154" distance of L0.end L18.end
  measures "d155" distance of L1.end L20.end
  measures "d156" distance of L1.end L21.start
  measures "d201" diameter of A5
  measures "d202" diameter of A6
  measures "d203" diameter of A7
  measures "d204" diameter of A8
extrude "Estrusione12" add sketch "Schizzo18" against normal blind 10 contours L0 L3 L12 L13 L14 L15 A6 | L0 L14 A6 | L3 L13 A6 | L0 L18 A7 | L2 L3 L8 L9 A5 | L0 L1 L16 L17 L18 L19 A7 | L1 L17 A7 | L1 L2 L20 L21 A8 | A4 bodies 1 in component "Cubo"
sketch "Schizzo19" plane through (0, 0, 101) normal (0, 0, -1) x (1, 0, 0) in component "Cubo"
  arc A0 (-33, -90) -> (-30, -87) centre (-33, -87) ccw
  line L0 (-30, -87) -> (-30, -3)
  arc A1 (-30, -3) -> (-33, 0) centre (-33, -3) ccw
  line L1 (-33, 0) -> (-117, 0)
  arc A2 (-117, 0) -> (-120, -3) centre (-117, -3) ccw
  line L2 (-120, -3) -> (-120, -87)
  arc A3 (-120, -87) -> (-117, -90) centre (-117, -87) ccw
  line L3 (-117, -90) -> (-33, -90)
  line L4 (-108, -12) -> (-116.5, -12)
  line L5 (-116.5, -12) -> (-116.5, -3.5)
  line L6 (-116.5, -3.5) -> (-108, -3.5)
  line L7 (-108, -3.5) -> (-108, -12)
  line L8 (-42, -12) -> (-33.5, -12)
  line L9 (-33.5, -12) -> (-33.5, -3.5)
  line L10 (-33.5, -3.5) -> (-42, -3.5)
  line L11 (-42, -3.5) -> (-42, -12)
  line L12 (-42, -78) -> (-33.5, -78)
  line L13 (-33.5, -78) -> (-33.5, -86.5)
  line L14 (-33.5, -86.5) -> (-42, -86.5)
  line L15 (-42, -86.5) -> (-42, -78)
  line L16 (-108, -78) -> (-116.5, -78)
  line L17 (-116.5, -78) -> (-116.5, -86.5)
  line L18 (-116.5, -86.5) -> (-108, -86.5)
  line L19 (-108, -86.5) -> (-108, -78)
  line L20 (-33.5, -13.5) -> (-33.5, -76.5)
  arc A4 (-33.5, -76.5) -> (-43.5, -86.5) centre (-33.5, -86.5) ccw
  line L21 (-43.5, -86.5) -> (-106.5, -86.5)
  arc A5 (-106.5, -86.5) -> (-116.5, -76.5) centre (-116.5, -86.5) ccw
  line L22 (-116.5, -76.5) -> (-116.5, -13.5)
  arc A6 (-116.5, -13.5) -> (-106.5, -3.5) centre (-116.5, -3.5) ccw
  line L23 (-106.5, -3.5) -> (-43.5, -3.5)
  arc A7 (-43.5, -3.5) -> (-33.5, -13.5) centre (-33.5, -3.5) ccw
  line L24 (-33.5, -76.5) -> (-33.5, -86.5)
  line L25 (-43.5, -86.5) -> (-33.5, -86.5)
  line L26 (-43.5, -3.5) -> (-33.5, -3.5)
  line L27 (-33.5, -13.5) -> (-33.5, -3.5)
  line L28 (-106.5, -3.5) -> (-116.5, -3.5)
  line L29 (-116.5, -3.5) -> (-116.5, -13.5)
  line L30 (-116.5, -76.5) -> (-116.5, -86.5)
  line L31 (-116.5, -86.5) -> (-106.5, -86.5)
  dimension "d159" = 8.5
  dimension "d160" = 8.5
  dimension "d161" = 8.5
  dimension "d162" = 8.5
  dimension "d163" = 8.5
  dimension "d164" = 8.5
  dimension "d165" = 8.5
  dimension "d166" = 8.5
  constraint horizontal L4
  constraint vertical L5
  constraint horizontal L6
  constraint vertical L7
  constraint horizontal L8
  constraint vertical L9
  constraint horizontal L10
  constraint vertical L11
  constraint horizontal L12
  constraint vertical L13
  constraint horizontal L14
  constraint vertical L15
  constraint horizontal L16
  constraint vertical L17
  constraint horizontal L18
  constraint vertical L19
  constraint coincident L20.end A4.start
  constraint perpendicular L14 L24
  constraint coincident A4.end L21.start
  constraint perpendicular L24 L25
  constraint coincident L23.end A7.start
  constraint perpendicular L9 L26
  constraint coincident L20.start A7.end
  constraint coincident L9.end L10.start
  constraint coincident A6.end L23.start
  constraint coincident L5.end L6.start
  constraint coincident L22.end A6.start
  constraint coincident A5.end L22.start
  constraint perpendicular L18 L30
  constraint coincident L21.end A5.start
  constraint perpendicular L19 L31
  measures "d159" distance of L4.start L4.end
  measures "d160" distance of L4.start L6.end
  measures "d161" distance of L8.start L8.end
  measures "d162" distance of L8.start L10.end
  measures "d163" distance of L12.start L12.end
  measures "d164" distance of L12.start L14.end
  measures "d165" distance of L16.start L16.end
  measures "d166" distance of L16.start L18.end
extrude "Estrusione13" cut sketch "Schizzo19" against normal blind 5 contours L4 A6 L29 | L4 L5 L6 L7 A6 L28 L29 | L7 A6 L28 | L16 A5 L30 | L11 A7 L26 | L16 L17 L18 L19 A5 L30 L31 | L8 L9 L10 L11 A7 L26 L27 | L19 A5 L31 | L8 A7 L27 | L15 A4 L25 | L12 A4 L24 | L12 L13 L14 L15 A4 L24 L25 bodies 1 in component "Cubo"
sketch "Schizzo20" plane through (0, 0, 106) normal (0, 0, -1) x (1, 0, 0) in component "Cubo"
  line L0 (-33.5, -13.5) -> (-33.5, -3.5)
  line L1 (-33.5, -3.5) -> (-43.5, -3.5)
  circle A0 centre (-112, -8) radius 2.75
  line L2 (-33, 0) -> (-117, 0)
  line L3 (-120, -3) -> (-120, -87)
  line L4 (-75, 0) -> (-75, 5)
  line L5 (-120, -45) -> (-127, -45)
  circle A1 centre (-38, -8) radius 2.75
  circle A2 centre (-112, -82) radius 2.75
  circle A3 centre (-38, -82) radius 2.75
  arc A4 (-43.5, -3.5) -> (-33.5, -13.5) centre (-33.5, -3.5) ccw
  dimension "d169" = 5.5
  dimension "d170" = 8
  dimension "d171" = 8
  constraint midpoint L2 L4.start
  constraint perpendicular L2 L4
  constraint midpoint L3 L5.start
  constraint perpendicular L3 L5
  constraint symmetric A0 L4 A1
  constraint symmetric A0 L5 A2
  constraint symmetric L5 A1 A3
  measures "d169" diameter of A0
  measures "d170" distance of A0.centre L2
  measures "d171" distance of A0.centre L3
extrude "Estrusione14" cut sketch "Schizzo20" against normal blind 1.5 contours A0 | A1 | A2 | A3 bodies 1 in component "Cubo"
copy_body "Corpo->Comp1" bodies 1 removing the originals makes body 3 in component "Coperchio"
fillet "Raccordo1'" radius 1 31 edges at (-85, 1, 148.5858) (-85.7929, 1, 142.2929) (-95, 1, 141.5) (-75, 1, 154.5) (-84.7929, 1, 154.2929) (-59.0858, 1, 129.5) (-64.7929, 1, 129.2929) (-65, 1, 124.3358) (-49.2929, 1, 133.7929) (-45, 1, 149) (-65.7929, 1, 118.7929) (-75, 1, 118) (-65, 1, 109) (-65.7929, 1, 102.7929) (-75, 1, 102) (-85, 1, 109) (-84.2071, 1, 102.7929) (-85, 1, 127.25) (-84.2071, 1, 118.7929) (-65, 1, 149) (-65.2071, 1, 154.2929) (-105, 1, 151.5) (-104.2071, 1, 142.2929) (-80.7071, 1, 139.2071) (-70.9142, 1, 143.5) (-100.7071, 1, 164.2071) (-75, 1, 168.5) (-84.2071, 1, 115.2071) (-75, 1, 116) (-65.7929, 1, 115.2071) (-49.2929, 1, 164.2071) on bodies 3 in component "Coperchio"
fillet "Raccordo2'" radius 1 33 edges at (-31, 55, 124.3358) (-31, 54.2071, 118.7929) (-31, 45, 118) (-31, 60.9142, 129.5) (-31, 55.2071, 129.2929) (-31, 70.7071, 133.7929) (-31, 75, 149) (-31, 35, 148.5858) (-31, 34.2071, 142.2929) (-31, 25, 141.5) (-31, 45, 154.5) (-31, 35.2071, 154.2929) (-31, 54.2071, 102.7929) (-31, 55, 109) (-31, 45, 102) (-31, 35, 127.25) (-31, 35.7929, 118.7929) (-31, 35, 109) (-31, 35.7929, 102.7929) (-31, 54.7929, 154.2929) (-75, 3.5, 101) (-31, 55, 149) (-31, 15.7929, 142.2929) (-31, 15, 151.5) (-31, 45, 168.5) (-31, 19.2929, 164.2071) (-31, 54.7929, 143.7071) (-31, 49.0858, 143.5) (-31, 39.2929, 139.2071) (-31, 45, 116) (-31, 35.7929, 115.2071) (-31, 54.2071, 115.2071) (-31, 70.7071, 164.2071) on bodies 3 in component "Coperchio"
fillet "Raccordo3" radius 1 32 edges at (-85, 89, 124.3358) (-84.2071, 89, 118.7929) (-75, 89, 118) (-90.9142, 89, 129.5) (-85.2071, 89, 129.2929) (-100.7071, 89, 133.7929) (-105, 89, 149) (-85, 89, 109) (-84.2071, 89, 102.7929) (-75, 89, 102) (-65, 89, 148.5858) (-64.2071, 89, 142.2929) (-55, 89, 141.5) (-75, 89, 154.5) (-65.2071, 89, 154.2929) (-45, 89, 151.5) (-45.7929, 89, 142.2929) (-65, 89, 127.25) (-65.7929, 89, 118.7929) (-65, 89, 109) (-65.7929, 89, 102.7929) (-85, 89, 149) (-84.7929, 89, 154.2929) (-84.7929, 89, 143.7071) (-79.0858, 89, 143.5) (-69.2929, 89, 139.2071) (-49.2929, 89, 164.2071) (-75, 89, 168.5) (-75, 89, 116) (-65.7929, 89, 115.2071) (-84.2071, 89, 115.2071) (-100.7071, 89, 164.2071) on bodies 3 in component "Coperchio"
fillet "Raccordo4" radius 1 32 edges at (-119, 74.2071, 142.2929) (-119, 75, 151.5) (-119, 65, 141.5) (-119, 35.2071, 154.2929) (-119, 45, 154.5) (-119, 35, 149) (-119, 55, 127.25) (-119, 54.2071, 118.7929) (-119, 45, 118) (-119, 55, 109) (-119, 54.2071, 102.7929) (-119, 45, 102) (-119, 29.0858, 129.5) (-119, 55, 148.5858) (-119, 55.7929, 142.2929) (-119, 15, 149) (-119, 19.2929, 133.7929) (-119, 35, 109) (-119, 35.7929, 102.7929) (-119, 35, 124.3358) (-119, 35.7929, 118.7929) (-119, 34.7929, 129.2929) (-119, 54.7929, 154.2929) (-119, 45, 116) (-119, 35.7929, 115.2071) (-119, 40.9142, 143.5) (-119, 45, 168.5) (-119, 19.2929, 164.2071) (-119, 70.7071, 164.2071) (-119, 35.2071, 143.7071) (-119, 50.7071, 139.2071) (-119, 54.2071, 115.2071) on bodies 3 in component "Coperchio"